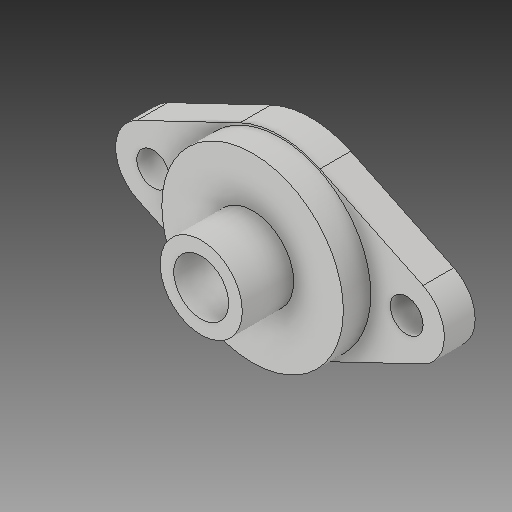
# Autodesk Inventor part: KFL08
Saved by Autodesk Inventor 2017 (Build 210142000, 142)
## iProperties
Part Number: KFL08
Material: Типовые
Document SubType Name: Modeling
Designer: Daemon
Density: 1 g/cm^3
Appearance: По умолчанию
Author: Daemon
Autodesk Inventor part; units mm, degrees
ref_plane "YZ Plane" through (0, 0, 0) normal (1, 0, 0) x (0, 1, 0)
ref_plane "XZ Plane" through (0, 0, 0) normal (0, 1, 0) x (-1, 0, 0)
ref_plane "XY Plane" through (0, 0, 0) normal (0, 0, 1) x (1, 0, 0)
sketch "Эскиз1" plane through (0, 0, 0) normal (0, 0, 1) x (1, 0, 0)
  arc A0 (4, 0) -> (-4, 0) centre (0, 0) ccw
  arc A1 (-16.1, 0) -> (-20.9, 0) centre (-18.5, 0) ccw
  arc A2 (20.9, 0) -> (16.1, 0) centre (18.5, 0) ccw
  line L0 (-24, 0) -> (24, 0)
  line L1 (-20.8784, 4.9592) -> (-5.8378, 12.1725)
  line L2 (20.8784, 4.9592) -> (5.8378, 12.1725)
  arc A3 (-20.8784, 4.9592) -> (-24, 0) centre (-18.5, 0) ccw
  arc A4 (24, 0) -> (20.8784, 4.9592) centre (18.5, 0) ccw
  arc A5 (5.8378, 12.1725) -> (-5.8378, 12.1725) centre (0, 0) ccw
  dimension "d0" = 8
  dimension "d9" = 37
  dimension "d12" = 4.8
  dimension "d14" = 48
  dimension "d15" = 5.5
  dimension "d16" = 13.5
  dimension "d19" = 0
  constraints: 12 point on circle, 6 centre point, 6 end point, 6 point on line, 4 coincident, 4 tangent, 2 equal radius, 1 equal length, 1 horizontal
  measures "d0" diameter of A0
  measures "d9" distance of A1.centre A2.centre
  measures "d12" diameter of A1
  measures "d14" distance of L0.start L0.end
  measures "d15" radius of A4
  measures "d16" radius of A5
  measures "d19" distance from line of point (0, 0) L0
extrude "Выдавливание1" add sketch "Эскиз1" along normal blind 4.5 contours A0 L0 A1 A3 L1 A5 L2 A4 A2
mirror "Зеркальное отражение1" about plane through (-24, 0, 0) normal (0, -1, 0) of "Выдавливание1"
sketch "Эскиз2" plane through (0, 0, 4.5) normal (0, 0, 1) x (1, 0, 0)
  circle A0 centre (0, 0) radius 4
  circle A1 centre (0, 0) radius 13.25
  dimension "d23" = 8
  dimension "d24" = 26.5
  constraints: 2 centre point, 2 coincident
  measures "d23" diameter of A0
  measures "d24" diameter of A1
extrude "Выдавливание2" add sketch "Эскиз2" along normal blind 4
sketch "Эскиз5" plane through (0, 0, 8.5) normal (0, 0, 1) x (1, 0, 0)
  circle A0 centre (0, 0) radius 6
  circle A1 centre (0, 0) radius 4
  dimension "d33" = 12
  dimension "d34" = 8
  constraints: 2 centre point, 2 coincident
  measures "d33" diameter of A0
  measures "d34" diameter of A1
extrude "Выдавливание5" add sketch "Эскиз5" along normal blind 7.5
